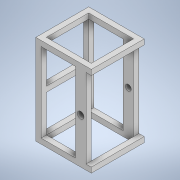
# Autodesk Inventor part: Glock Frame
Saved by Autodesk Inventor 2020 (Build 240168000, 168)
## iProperties
Created: 2020-02-15
Part Number: Glock Frame
Material: Generic
Document SubType Name: Modeling
Designer: aidan
Density: 1 g/cm^3
Appearance: Default
Author: aidan
Autodesk Inventor part; units mm, degrees
ref_plane "YZ Plane" through (0, 0, 0) normal (1, 0, 0) x (0, 1, 0)
ref_plane "XZ Plane" through (0, 0, 0) normal (0, 1, 0) x (-1, 0, 0)
ref_plane "XY Plane" through (0, 0, 0) normal (0, 0, 1) x (1, 0, 0)
sketch "Sketch1" plane through (0, 0, 0) normal (1, 0, 0) x (0, 1, 0)
  line L0 (130.5367, 151.1139) -> (-301.2633, 151.1139)
  line L1 (-301.2633, 151.1139) -> (-301.2633, -102.8861)
  line L2 (-301.2633, -102.8861) -> (130.5367, -102.8861)
  line L3 (130.5367, -102.8861) -> (130.5367, 151.1139)
  line L4 (105.1367, 125.7139) -> (-275.8633, 125.7139)
  line L5 (-275.8633, 125.7139) -> (-275.8633, -77.4861)
  line L6 (-275.8633, -77.4861) -> (105.1367, -77.4861)
  line L7 (105.1367, -77.4861) -> (105.1367, 125.7139)
  point P0 (0, 0)
  dimension "d0" = 254
  dimension "d1" = 431.8
  dimension "d2" = 25.4
  constraints: 16 end point, 4 parallel, 2 perpendicular, 1 horizontal, 3 other
  measures "d0" distance of L2.end L0.start
  measures "d1" distance of L1.end L2.end
  measures "d2" distance between parallel lines of L3 L7
extrude "Extrusion1" add sketch "Sketch1" along normal blind 266.7
sketch "Sketch2" plane through (0, -301.2633, 151.1139) normal (0, 0, 1) x (1, 0, 0)
  line L0 (0, 431.8) -> (0, 0) projected
  line L1 (0, 0) -> (266.7, 0) projected
  line L2 (266.7, 431.8) -> (266.7, 0) projected
  line L3 (0, 431.8) -> (266.7, 431.8) projected
  line L4 (190.5, 25.4) -> (25.4, 25.4)
  line L5 (25.4, 25.4) -> (25.4, 406.4)
  line L6 (25.4, 406.4) -> (190.5, 406.4)
  line L7 (190.5, 406.4) -> (190.5, 25.4)
  line L8 (0, 25.4) -> (266.7, 25.4) projected
  line L9 (266.7, 406.4) -> (241.3, 406.4)
  line L10 (241.3, 406.4) -> (241.3, 25.4)
  line L11 (241.3, 25.4) -> (266.7, 25.4)
  line L12 (266.7, 25.4) -> (266.7, 406.4)
  point P0 (0, 301.2633)
  dimension "d19" = 25.4
  dimension "d20" = 76.2
  dimension "d29" = 25.4
  constraints: 16 end point, 2 parallel, 2 point on line, 1 collinear, 1 horizontal, 1 perpendicular, 1 vertical, 2 other
  measures "d19" distance between parallel lines of L3 L6
  measures "d20" distance from line of L2 L6.end
  measures "d29" distance of L9.start L9.end
extrude "Extrusion2" cut sketch "Sketch2" against normal through all contours L5 L6 L7 L4 | L2 L8 L10 L9
sketch "Sketch3" plane through (0, 130.5367, 151.1139) normal (0, 1, 0) x (1, 0, 0)
  line L0 (0, 254) -> (0, 0) projected
  line L1 (0, 0) -> (266.7, 0) projected
  line L2 (266.7, 254) -> (266.7, 0) projected
  line L3 (0, 254) -> (266.7, 254) projected
  line L4 (25.4, 25.4) -> (25.4, 228.6)
  line L5 (25.4, 228.6) -> (241.3, 228.6)
  line L6 (241.3, 228.6) -> (241.3, 25.4)
  line L7 (241.3, 25.4) -> (25.4, 25.4)
  point P0 (0, 151.1139)
  dimension "d8" = 25.4
  constraints: 8 end point, 3 other
  measures "d8" distance between parallel lines of L0 L4
extrude "Extrusion3" cut sketch "Sketch3" against normal through all contours L4 L5 L6 L7
sketch "Sketch4" plane through (0, -275.8633, -77.4861) normal (0, 0, 1) x (1, 0, 0)
  line L0 (25.4, 381) -> (25.4, 0) projected
  line L1 (25.4, 0) -> (25.4, 381) projected
  line L2 (25.4, 177.8) -> (0, 177.8)
  line L3 (0, 177.8) -> (0, 203.2)
  line L4 (0, 203.2) -> (25.4, 203.2)
  line L5 (25.4, 203.2) -> (25.4, 177.8)
  point P0 (0, 275.8633)
  point P1 (0, -17.3634)
  point P2 (0, 0)
  point P3 (0, 381)
  dimension "d13" = 25.4
  dimension "d15" = 177.8
  dimension "d16" = 177.8
  constraints: 8 end point, 2 parallel, 1 horizontal, 1 perpendicular, 1 point on line
  measures "d13" distance of L3.end L4.end
  measures "d15" distance from line of L2 point (0, 0)
  measures "d16" distance from line of point (0, 381) L4
extrude "Extrusion4" add sketch "Sketch4" along normal up to surface (203.2 mm away)
sketch "Sketch7" plane through (0, -301.2633, 151.1139) normal (0, 0, 1) x (1, 0, 0)
  circle A0 centre (215.9, 215.9) radius 15.875
  line L0 (241.3, 25.4) -> (241.3, 406.4) projected
  line L1 (0, 0) -> (266.7, 0) projected
  point P0 (0, 301.2633)
  dimension "d30" = 31.75
  dimension "d31" = 25.4
  dimension "d32" = 215.9
  constraints: 1 centre point
  measures "d30" diameter of A0
  measures "d31" distance from line of L0 A0.centre
  measures "d32" distance from line of L1 A0.centre
extrude "Extrusion7" cut sketch "Sketch7" against normal blind 25.4
sketch "Sketch8" plane through (190.5, -275.8633, -77.4861) normal (0, 0, 1) x (1, 0, 0)
  circle A0 centre (25.4, 190.5) radius 15.875 projected
  circle A1 centre (25.4, 190.5) radius 14.2875
  point P0 (-190.5, 275.8633)
  dimension "d35" = 28.575
  constraints: 1 centre point, 1 coincident
  measures "d35" diameter of A1
extrude "Extrusion8" cut sketch "Sketch8" against normal blind 25.4 contours A1
body "Solid1"
